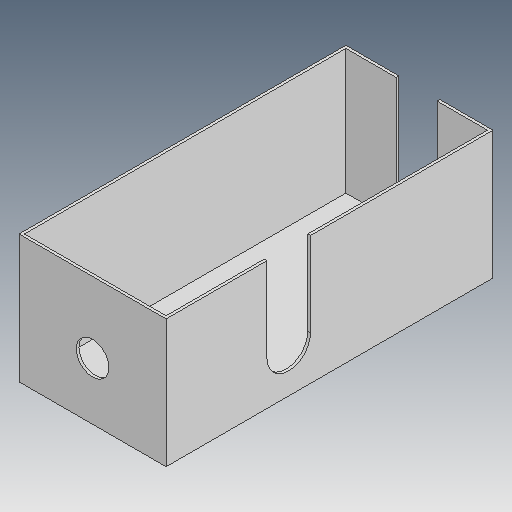
# Autodesk Inventor part: tension_sensor_cover
Saved by Autodesk Inventor 2025.2 (Build 292293000, 293)
## iProperties
Created: 2025-02-17
Part Number: tension_sensor_cover
Material: Generic
Document SubType Name: Modeling
Designer: email
Density: 1 g/cm^3
Appearance: Default
Author: email
Autodesk Inventor part; units mm, degrees
ref_plane "YZ Plane" through (0, 0, 0) normal (1, 0, 0) x (0, 1, 0)
ref_plane "XZ Plane" through (0, 0, 0) normal (0, 1, 0) x (-1, 0, 0)
ref_plane "XY Plane" through (0, 0, 0) normal (0, 0, 1) x (1, 0, 0)
sketch "Sketch1" plane through (0, 0, 0) normal (0, 1, 0) x (-1, 0, 0)
  line L0 (0, 0) -> (-54, 0)
  line L1 (-54, 0) -> (-54, -120)
  line L2 (-54, -120) -> (0, -120)
  line L3 (0, -120) -> (0, 0)
  line L4 (-1, -1) -> (-53, -1)
  line L5 (-53, -1) -> (-53, -119)
  line L6 (-53, -119) -> (-34.5, -119)
  line L7 (-34.5, -119) -> (-34.5, -120)
  line L8 (-1, -1) -> (-1, -119)
  line L9 (-1, -119) -> (-19.5, -119)
  line L10 (-19.5, -119) -> (-19.5, -120)
  dimension "d0" = 54
  dimension "d1" = 120
  dimension "d2" = 1
  dimension "d3" = 1
  dimension "d4" = 1
  dimension "d5" = 1
  dimension "d6" = 15
  constraints: 22 end point, 6 perpendicular, 2 collinear, 2 horizontal, 2 parallel, 2 point on line, 1 vertical
  measures "d0" distance of L0.start L0.end
  measures "d1" distance of L0.end L1.end
  measures "d2" distance between parallel lines of L3 L8
  measures "d3" distance between parallel lines of L1 L5
  measures "d4" distance between parallel lines of L0 L4
  measures "d5" distance between parallel lines of L2 L9
  measures "d6" distance between parallel lines of L7 L10
extrude "Extrusion1" add sketch "Sketch1" against normal blind 1
extrude "Extrusion2" add sketch "Sketch1" along normal blind 46 contours L3 L2 L10 L9 L8 L4 L5 L6 L7 L1 L0
sketch "Sketch2" plane through (0, -1, 0) normal (0, 0, 1) x (1, 0, 0)
  circle A0 centre (27, 21) radius 6
  line L0 (0, 47) -> (54, 47) projected
  line L1 (54, 0) -> (54, 47) projected
  point P0 (0, 1)
  point P1 (27, 47)
  dimension "d11" = 26
  dimension "d12" = 12
  constraints: 1 centre point, 1 midpoint, 1 vertical alignment
  measures "d11" distance from line of L0 A0.centre
  measures "d12" diameter of A0
extrude "Extrusion3" cut sketch "Sketch2" against normal up to next
sketch "Sketch3" plane through (54, -1, 0) normal (1, 0, 0) x (0, 0, -1)
  arc A0 (37, 16) -> (53, 16) centre (45, 16) ccw
  line L0 (0, 0) -> (0, 47) projected
  line L1 (53, 16) -> (53, 47)
  line L2 (53, 47) -> (37, 47)
  line L3 (37, 47) -> (37, 16)
  line L4 (0, 47) -> (120, 47) projected
  point P0 (0, 1)
  dimension "d16" = 45
  dimension "d17" = 16
  dimension "d18" = 31
  constraints: 6 end point, 2 point on circle, 2 tangent, 1 centre point, 1 parallel, 1 perpendicular, 1 vertical
  measures "d16" distance from line of L0 A0.centre
  measures "d17" diameter of A0
  measures "d18" distance from line of L4 A0.centre
extrude "Extrusion4" cut sketch "Sketch3" against normal up to surface (1 mm away)
body "Solid1"
